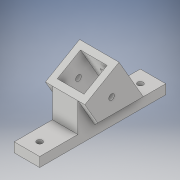
# Autodesk Inventor part: 60DegreeAttachementV03
Saved by Autodesk Inventor 2019.3 (Build 233278000, 278)
## iProperties
Created: 2019-02-16
Part Number: 60DegreeAttachementV03
Material: Generic
Document SubType Name: Modeling
Designer: steele
Density: 1 g/cm^3
Appearance: Default
Author: steele
Autodesk Inventor part; units mm, degrees
note: some values were not read from the file. Chosen so that the rebuilt part matches the saved one: direction of "Hole2".
ref_plane "YZ Plane" through (0, 0, 0) normal (1, 0, 0) x (0, 1, 0)
ref_plane "XZ Plane" through (0, 0, 0) normal (0, 1, 0) x (-1, 0, 0)
ref_plane "XY Plane" through (0, 0, 0) normal (0, 0, 1) x (1, 0, 0)
sketch "Sketch1" plane through (0, 0, 0) normal (1, 0, 0) x (0, 1, 0)
  line L0 (0, 0) -> (29.1856, 16.8503)
  line L1 (29.1856, 16.8503) -> (48.8706, -17.2451)
  line L2 (0, -71.1236) -> (0, 36.9987) projected
  line L3 (48.8706, -17.2451) -> (0, -45.4606)
  line L4 (0, 0) -> (0, -45.4606)
  line L5 (32.9956, 10.2512) -> (0, -8.7988) construction
  dimension "d0" = 39.37
  dimension "d1" = 60
  dimension "d5" = 7.62
  dimension "d6" = 38.1
  constraints: 10 end point, 3 point on line, 2 parallel, 1 collinear, 1 perpendicular
  measures "d0" distance of L0.end L1.end
  measures "d1" angle of L0 L2
  measures "d5" distance between parallel lines of L5 L0
  measures "d6" distance from line of L5.end L1
extrude "Extrusion1" add sketch "Sketch1" along normal mid plane 39.37
sketch "Sketch2" plane through (-19.685, 29.1856, 16.8503) normal (0, 0.8660254, 0.5) x (1, 0, 0)
  line L0 (0, 0) -> (39.37, 0) construction
  line L1 (39.37, 0) -> (39.37, 39.37) construction
  line L2 (0, 0) -> (39.37, 39.37) construction
  line L3 (39.37, 39.37) -> (0, 39.37) construction
  line L4 (0, 39.37) -> (39.37, 0) construction
  line L5 (6.35, 6.35) -> (33.02, 6.35)
  line L6 (33.02, 6.35) -> (33.02, 33.02)
  line L7 (33.02, 33.02) -> (6.35, 33.02)
  line L8 (6.35, 33.02) -> (6.35, 6.35)
  line L9 (6.35, 6.35) -> (33.02, 33.02) construction
  line L10 (33.02, 6.35) -> (6.35, 33.02) construction
  point P0 (19.685, 0)
  point P1 (19.685, 19.685)
  dimension "d7" = 26.67
  constraints: 16 end point, 3 midpoint, 2 parallel, 2 perpendicular, 1 horizontal
  measures "d7" distance of L7.end L5.start
extrude "Extrusion2" cut sketch "Sketch2" against normal blind 38.1
sketch "Sketch3" plane through (0, 0, 0) normal (1, 0, 0) x (0, 1, 0)
  line L0 (29.1856, 16.8503) -> (0, 0) projected
  line L1 (0, 0) -> (0, -45.4606) projected
  line L2 (0, -45.4606) -> (48.8706, -17.2451) projected
  line L3 (12.7, -30.7959) -> (0, -8.7988) projected
  line L4 (32.3606, 11.351) -> (0, -7.3323) projected
  line L5 (0, 0) -> (0, -45.4606)
  line L6 (29.1856, 16.8503) -> (15.6348, 16.8503) construction
  line L7 (0, 0) -> (29.1856, 16.8503) projected
  line L8 (0, 0) -> (0, 54.9503)
  line L9 (48.8706, -17.2451) -> (0, -45.4606) projected
  line L10 (0, -45.4606) -> (0, -70.8606)
  line L11 (0, -109.2236) -> (0, 87.7987) projected
  line L12 (0, 54.9503) -> (-9.525, 54.9503)
  line L13 (-9.525, 54.9503) -> (-9.525, -70.8606)
  line L14 (-9.525, -70.8606) -> (0, -70.8606)
  point P0 (1.0999, -13.335)
  point P1 (0, -15.24)
  point P2 (0, -8.7988)
  dimension "d10" = 38.1
  dimension "d11" = 25.4
  dimension "d12" = 9.525
  dimension "supportBaseLength" = 125.8109
  constraints: 14 end point, 5 vertical, 2 horizontal, 2 perpendicular, 3 other
  measures "d10" distance from line of L8.end L6
  measures "d11" distance of L1.end L10.end
  measures "d12" distance of L8.end L12.end
  measures "supportBaseLength" distance between parallel lines of L14 L12
extrude "Extrusion3" add sketch "Sketch3" along normal mid plane 25.4
sketch "Sketch5" plane through (0, 0, 0) normal (1, 0, 0) x (0, 1, 0)
  line L0 (0, 0) -> (29.1856, 16.8503) projected
  line L1 (0, 54.9503) -> (0, 0) projected
  line L2 (29.1856, 16.8503) -> (48.8706, -17.2451) projected
  line L3 (29.1856, 16.8503) -> (0, 16.8503)
  line L4 (0, 0) -> (29.1856, 16.8503)
  constraints: 4 end point, 1 horizontal, 1 point on line
extrude "Extrusion5" add sketch "Sketch5" along normal mid plane 25.4
sketch "Sketch4" plane through (0, 0, 0) normal (0, 0, 1) x (1, 0, 0)
  line L0 (19.685, 48.8706) -> (-19.685, 48.8706) projected
  line L1 (19.685, 0) -> (19.685, 48.8706) projected
  line L2 (19.685, 0) -> (12.7, 0) projected
  line L3 (12.7, 0) -> (-12.7, 0) projected
  line L4 (-12.7, 0) -> (-19.685, 0) projected
  line L5 (-19.685, 48.8706) -> (-19.685, 0) projected
  line L6 (-12.7, 0) -> (-12.7, -9.525) projected
  line L7 (12.7, -9.525) -> (-12.7, -9.525) projected
  line L8 (12.7, -9.525) -> (12.7, 0) projected
  line L9 (-12.7, 0) -> (-19.685, 6.985)
  line L10 (-19.685, 48.8706) -> (-19.685, 0) projected
  line L11 (-19.685, 6.985) -> (-19.685, 0)
  line L12 (0, 0) -> (0, 48.8706) construction
  line L13 (12.7, 0) -> (19.685, 0)
  line L14 (12.7, 0) -> (19.685, 6.985)
  line L15 (19.685, 6.985) -> (19.685, 0)
  dimension "d15" = 45
  constraints: 12 end point, 1 collinear, 1 midpoint, 1 point on line, 1 symmetric about line
  measures "d15" angle of L9 L4
extrude "Extrusion4" cut sketch "Sketch4" against normal up to surface (125.8109 mm away) from surface at 54.9503 contours L1 L2 L14 | L9 L4 L5
sketch "Sketch6" plane through (-12.7, 0, 54.9503) normal (0, 1, 0) x (1, 0, 0)
  line L0 (25.4, 125.8109) -> (0, 125.8109) construction
  line L1 (12.7, 125.8109) -> (12.7, 0) construction
  line L2 (25.4, 0) -> (0, 0) construction
  point P0 (12.7, 54.9503)
  point P1 (12.7, 113.1109)
  point P2 (12.7, 12.7)
  dimension "d21" = 12.7
  dimension "d22" = 12.7
  constraints: 2 end point, 2 midpoint, 2 point on line
  measures "d21" distance from line of point (12.7, 12.7) L2
  measures "d22" distance from line of point (12.7, 113.111) L0
hole "Hole1" at (0, 0, -58.1606) at (0, 0, 42.2503) direction (0, -1, 0) diameter 5.6134 end through all clearance for "Flat Head Machine Screw (82)" size "#10" standard "Ansi Unified Screw Threads"
sketch "Sketch9" plane through (0, 0, 0) normal (1, 0, 0) x (0, 1, 0)
  line L0 (0.635, -6.9657) -> (0.635, -9.8987) projected
  line L1 (0.635, -9.8987) -> (12.7, -30.7959) projected
  line L2 (45.6956, -11.7459) -> (12.7, -30.7959) projected
  line L3 (32.3606, 11.351) -> (45.6956, -11.7459) projected
  line L4 (32.3606, 11.351) -> (0.635, -6.9657) projected
  line L5 (39.0281, -0.1974) -> (6.0325, -19.2474) construction
  line L6 (0.635, -9.8987) -> (12.7, -30.7959) construction
  circle A0 centre (22.5303, -9.7224) radius 2.8067
  point P0 (0, 0)
  dimension "d30" = 5.6134
  constraints: 2 end point, 2 midpoint, 1 centre point, 1 perpendicular, 1 point on line
  measures "d30" diameter of A0
extrude "Extrusion6" cut sketch "Sketch9" along normal through all both and the other way through all contours A0
sketch "Sketch10" plane through (-19.685, 48.8706, -17.2451) normal (0, 0.5, -0.8660254) x (1, 0, 0)
  line L0 (6.35, 0) -> (33.02, 0) construction
  line L1 (19.685, 0) -> (19.685, 77.7875) construction
  point P0 (19.685, 33.7006)
  point P1 (19.685, 19.05)
  dimension "d33" = 19.05
  constraints: 2 end point, 1 midpoint, 1 point on line, 1 vertical
  measures "d33" distance from line of point (19.685, 19.05) L0
hole "Hole2" at (0, 32.3728, -26.7701) direction (0, -0.5, 0.8660254) diameter 5.6134 depth 6.35 clearance for "Flat Head Machine Screw (82)" size "#10" standard "Ansi Unified Screw Threads"
equation "\"d0\" = widthToSupportExtrusion"
equation "\"d1\" = attachementAngle"
equation "\"d6\" = insertDepth"
equation "\"d2\" = widthToSupportExtrusion"
equation "\"d7\" = insertForExtrusion"
equation "\"d8\" = insertDepth"
equation "\"d10\" = lenghtUnderBrace"
equation "\"d11\" = backLength"
equation "\"d12\" = supportBaseDepth"
equation "\"d13\" = supportBaseWidth"
equation "\"d19\" = supportBaseWidth"
equation "\"d21\" = supportHoleDistanceFromEnd"
equation "\"d22\" = supportHoleDistanceFromEnd"
equation "\"attachementAngle\" = 60deg"
equation "\"extrusionSize\" = 25.4"
equation "\"wallThickness\" = 6.35"
equation "\"slipClearance\" = 0.635"
equation "\"insertForExtrusion\" = extrusionSize + 2 * slipClearance"
equation "\"widthToSupportExtrusion\" = insertForExtrusion + 2 * wallThickness"
equation "\"insertDepth\" = 38.1"
equation "\"supportBaseWidth\" = 25.4"
equation "\"supportBaseDepth\" = 9.525"
equation "\"supportHoleDistanceFromEnd\" = 12.7"
equation "\"lenghtUnderBrace\" = 38.1"
equation "\"backLength\" = 25.4"
body "Solid1"
